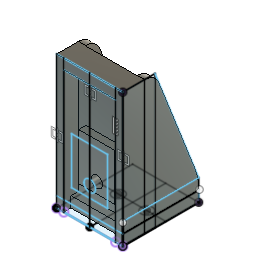
sensor_holder (Autodesk Fusion 360 design; units mm, degrees)
Autodesk Fusion 360 part; units mm, degrees
note: some values were not read from the file. Set by a fixed rule: which sketch regions a step uses.
sketch "vertical plane" plane through (0, 0, 0) normal (0, 1, 0) x (-1, 0, 0)
  circle A0 centre (0, 10) radius 1.6
  line L0 (-7.25, 0) -> (7.25, 0)
  line L1 (7.25, 0) -> (7.25, 37.31)
  line L2 (7.25, 37.31) -> (-7.25, 37.31)
  line L3 (-7.25, 37.31) -> (-7.25, 0)
  line L4 (0, 0) -> (0, 37.31)
  line L5 (-9.25, 0) -> (9.25, 0)
  line L6 (9.25, 0) -> (9.25, 37.3146)
  line L7 (9.25, 37.3146) -> (-9.25, 37.3146)
  line L8 (-9.25, 37.3146) -> (-9.25, 0)
  line L9 (-9.25, 3) -> (9.25, 3)
  line L10 (-7.25, 34.5) -> (7.25, 34.5)
  line L11 (-4.9614, 7) -> (5.0877, 7)
  line L12 (5.0877, 7) -> (5.0877, 20.0804)
  line L13 (5.0877, 20.0804) -> (-4.9614, 20.0804)
  line L14 (-4.9614, 20.0804) -> (-4.9614, 7)
  dimension "d43" = 3.2
  dimension "d72" = 14.5
  dimension "d73" = 2
  dimension "d74" = 3
  dimension "d75" = 31.5
  dimension "d76" = 7
  dimension "d77" = 4
  constraint horizontal L0
  constraint vertical L1
  constraint horizontal L2
  constraint vertical L3
  constraint coincident L4.start origin
  constraint coincident L2 L4.end
  constraint perpendicular L2 L4
  constraint symmetric L1 L3 L4
  constraint coincident A0.centre L4
  constraint horizontal L5
  constraint vertical L6
  constraint horizontal L7
  constraint vertical L8
  constraint symmetric L4 L6 L8
  constraint coincident L8 L9.start
  constraint coincident L6 L9.end
  constraint perpendicular L6 L9
  constraint coincident L3 L10.start
  constraint coincident L1 L10.end
  constraint perpendicular L1 L10
  constraint horizontal L11
  constraint vertical L12
  constraint horizontal L13
  constraint vertical L14
  constraint collinear L0 L5
  measures "d43" diameter of A0
  measures "d72" distance of L0.start L0.end
  measures "d73" distance of L3 L8
  measures "d74" distance of L5 L9
  measures "d75" distance of L9 L10
  measures "d76" distance of A0.centre L9
  measures "d77" distance of L9 L11
sketch "Sketch25" plane through (0, 0, 0) normal (0, 0, 1) x (1, 0, 0)
  line L0 (9.25, 0) -> (-9.25, 0)
  line L1 (9.25, 0) -> (9.25, 21.23)
  line L2 (9.25, 21.23) -> (-9.25, 21.23)
  line L3 (-9.25, 21.23) -> (-9.25, 0)
  line L4 (-9.25, 12) -> (9.25, 12)
  line L5 (0, 21.23) -> (0, 0)
  line L6 (9.25, 0) -> (-9.25, 0)
  circle A0 centre (-4, 12) radius 1.575
  circle A1 centre (4, 12) radius 1.575
  point P0 (7.25, 0)
  point P1 (9.25, 0)
  point P2 (-7.25, 0)
  point P3 (-9.25, 0)
  dimension "d112" = 21.23
  dimension "d113" = 12
  dimension "d114" = 3.15
  dimension "d115" = 3.15
  dimension "d116" = 8
  constraint coincident P3 L0.end
  constraint horizontal L0
  constraint coincident P1 L0.start
  constraint parallel L1 L3
  constraint coincident L3 L4.start
  constraint coincident L1 L4.end
  constraint perpendicular L1 L4
  constraint midpoint L2 L5.start
  constraint coincident L5.end origin
  constraint perpendicular L0 L5
  constraint coincident L4 A0.centre
  constraint coincident L4 A1.centre
  constraint symmetric L5 A0 A1
  constraint parallel L2 L6
  measures "d112" distance of P3 L2.end
  measures "d113" distance of L4 L6
  measures "d114" diameter of A0
  measures "d115" diameter of A1
  measures "d116" distance of A0.centre A1.centre
ref_plane "WorkPlane2" through (9.25, 0, 18.6573) normal (-1, 0, 0) x (0, 0, -1)
sketch "side plane details" plane through (9.25, 0, 0) normal (-1, 0, 0) x (0, -1, 0)
  line L0 (0, 0) -> (-21.2275, 0)
  line L1 (-21.2275, 0) -> (-21.2275, 3)
  line L2 (-21.2275, 3) -> (0, 3)
  line L3 (0, 3) -> (0, 0)
  line L4 (0, 37.3146) -> (-9, 37.3146)
  line L5 (-9, 37.3146) -> (-9, 0)
  line L6 (-9, 0) -> (0, 0)
  line L7 (0, 0) -> (0, 37.3146)
  line L8 (-6, 0) -> (-6, 37.3146)
  line L9 (0, 3) -> (-21.4, 3)
  line L10 (0, 5.7) -> (0, 3)
  line L11 (-21.23, 0) -> (0, 0)
  line L12 (0, 0) -> (0, 5.9996)
  line L13 (0, 5.9996) -> (-21.23, 5.9996)
  line L14 (-21.23, 5.9996) -> (-21.23, 0)
  line L15 (-9, 37.3146) -> (-21.23, 5.9996)
  point P0 (0, 37.3146)
  point P1 (-21.23, 0)
  dimension "d83" = 9
  dimension "d84" = 3
  dimension "d89" = 6
  constraint horizontal L0
  constraint vertical L1
  constraint horizontal L2
  constraint vertical L3
  constraint coincident L0.start L3.end
  constraint horizontal L4
  constraint vertical L5
  constraint horizontal L6
  constraint vertical L7
  constraint coincident P0 L4.start
  constraint coincident L6 L8.start
  constraint coincident L0 L8.start
  constraint coincident L4 L8.end
  constraint perpendicular L4 L8
  constraint horizontal L9
  constraint vertical L10
  constraint perpendicular L11 L12
  constraint parallel L11 L13
  constraint parallel L12 L14
  constraint perpendicular L3 L11
  constraint coincident P1 L11.start
  measures "d83" distance of P0 L4.end
  measures "d84" distance of L0 L2
  measures "d89" distance of L7 L8
extrude "Extrude25" add sketch "Sketch25" along normal blind 3
extrude "Extrude26" add sketch "vertical plane" along normal blind 6
extrude "Extrude27" cut sketch "vertical plane" along normal blind 2 contours L0 L1 L4 L5 L9 | L0 L3 L4 L5 L9
extrude "Extrude28" cut sketch "vertical plane" along normal blind 4 contours A0 L4 | A0 L4 L11 L12 L13 | A0 L4 | A0 L4 L11 L13 L14 | L3 L4 L9 L10 L11 L13 L14 | L1 L4 L9 L10 L11 L12 L13
extrude "Extrude29" cut sketch "vertical plane" along normal blind 2 from surface at 4 contours A0 L4 | A0 L4
extrude "Extrude30" add sketch "vertical plane" against normal blind 2 from surface at 4 contours A0 L4 L11 L12 L13 | A0 L4 L11 L13 L14
extrude "Extrude31" cut sketch "Sketch25" along normal blind 3 contours L4 A1 | L4 A1 | L4 A0 | L4 A0
extrude "Extrude32" add sketch "side plane details" along normal blind 2 contours L2 L5 L8 L9 L13 | L2 L5 L9 L13 L14 | L4 L5 L8 L13 | L5 L13 L15
extrude "Extrude33" add 1 faces at (7.25, 12.0767, 15.4381) along direction (-1, 0, 0) blind 2 from surface at 14.5
fillet "Fillet1" radius 4.25 2 edges at (8.25, 9, 37.3146) (-8.25, 9, 37.3146)
fillet "Fillet2" radius 14.25 2 edges at (-8.25, 21.23, 5.9996) (8.25, 21.23, 5.9996)
